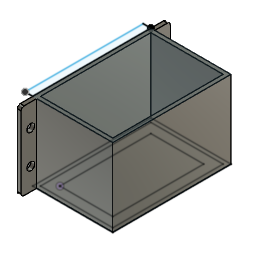
Housing_Power_Connector v1 (Autodesk Fusion 360 design; units mm, degrees)
Autodesk Fusion 360 part; units mm, degrees
sketch "Sketch1" plane through (0, 0, 0) normal (0, 0, 1) x (1, 0, 0)
  line L0 (0, 0) -> (27.2, 0)
  line L1 (27.2, 0) -> (27.2, 46.8)
  line L2 (27.2, 46.8) -> (0, 46.8)
  line L3 (0, 46.8) -> (0, 0)
  line L4 (-5, 51.8) -> (-5, -5)
  line L5 (-5, -5) -> (32.2, -5)
  line L6 (32.2, -5) -> (32.2, 51.8)
  line L7 (32.2, 51.8) -> (-5, 51.8)
  line L8 (-7, 53.8) -> (-7, -7)
  line L9 (-7, -7) -> (34.2, -7)
  line L10 (34.2, -7) -> (34.2, 53.8)
  line L11 (34.2, 53.8) -> (-7, 53.8)
  dimension "d1" = 27.2
  dimension "d2" = 46.8
  dimension "d3" = 5
  dimension "d4" = 7
  constraint horizontal L0
  constraint vertical L1
  constraint horizontal L2
  constraint vertical L3
  constraint coincident L0.start L3.end
  measures "d1" distance of L0.start L0.end
  measures "d2" distance of L0.start L2.end
extrude "Extrude1" add sketch "Sketch1" along normal blind 1.2 contours L4 L5 L6 L7
extrude "Extrude2" add sketch "Sketch1" along normal blind 40 contours L8 L9 L10 L11
sketch "Sketch2" plane through (0, 0, 40) normal (0, 0, 1) x (-1, 0, 0)
  line L0 (5, -51.8) -> (-32.2, -51.8)
  line L1 (-32.2, -51.8) -> (-32.2, 5)
  line L2 (-32.2, 5) -> (5, 5)
  line L3 (5, 5) -> (5, -51.8)
  line L4 (-34.2, -53.8) -> (7, -53.8)
  line L5 (7, -53.8) -> (7, 7)
  line L6 (7, 7) -> (-34.2, 7)
  line L7 (-34.2, 7) -> (-34.2, -53.8)
  line L8 (7, -53.8) -> (10.9437, -53.8)
  line L9 (10.9437, -53.8) -> (10.9437, 7)
  line L10 (10.9437, 7) -> (7, 7)
  line L11 (7, 7) -> (7, -53.8)
  constraint horizontal L8
  constraint vertical L9
  constraint horizontal L10
  constraint vertical L11
  constraint coincident L6 L9.end
  constraint coincident L4.end L5.start
sketch "Sketch3" plane through (0, -7, 0) normal (0, -1, 0) x (1, 0, 0)
  line L0 (-7, 0) -> (34.2, 0)
  line L1 (34.2, 0) -> (34.2, 40)
  line L2 (34.2, 40) -> (-7, 40)
  line L3 (-7, 40) -> (-7, 0)
  line L4 (-7, 0) -> (-5, 0)
  line L5 (-5, 0) -> (-5, 40)
  line L6 (-5, 40) -> (-7, 40)
  line L7 (-7, 40) -> (-7, 0)
  dimension "d9" = 2
  constraint horizontal L4
  constraint vertical L5
  constraint horizontal L6
  constraint vertical L7
  constraint coincident L2 L5.end
  constraint coincident L0.start L3.end
  measures "d9" distance of L0.start L4.end
extrude "Extrude3" add sketch "Sketch3" along normal blind 8 contours L0 L2 L3 L4 L5 L6 L7
sketch "Sketch4" plane through (0, 53.8, 0) normal (0, 1, 0) x (-1, 0, 0)
  line L0 (-34.2, 0) -> (7, 0)
  line L1 (7, 0) -> (7, 40)
  line L2 (7, 40) -> (-34.2, 40)
  line L3 (-34.2, 40) -> (-34.2, 0)
  line L4 (7, 0) -> (5, 0)
  line L5 (5, 0) -> (5, 40)
  line L6 (5, 40) -> (7, 40)
  line L7 (7, 40) -> (7, 0)
  dimension "d12" = 2
  constraint horizontal L4
  constraint vertical L5
  constraint horizontal L6
  constraint vertical L7
  constraint coincident L2 L5.end
  constraint coincident L0.end L1.start
  measures "d12" distance of L0.end L4.end
extrude "Extrude4" add sketch "Sketch4" along normal blind 8 contours L0 L1 L2 L4 L5 L6 L7
fillet "Fillet1" radius 1.5 4 edges at (-6, -15, 40) (-6, 61.8, 40) (-6, 61.8, 0) (-6, -15, 0)
sketch "Sketch5" plane through (-5, 0, 0) normal (1, 0, 0) x (0, 1, 0)
  arc A0 (60.3, 0) -> (61.8, 1.5) centre (60.3, 1.5) ccw
  line L0 (61.8, 1.5) -> (61.8, 38.5)
  arc A1 (61.8, 38.5) -> (60.3, 40) centre (60.3, 38.5) ccw
  line L1 (60.3, 40) -> (53.8, 40)
  line L2 (53.8, 40) -> (53.8, 0)
  line L3 (53.8, 0) -> (60.3, 0)
  line L4 (61.8, 11.3134) -> (-15, 11.3134) construction
  line L5 (61.8, 28.4248) -> (-15, 28.4248) construction
  line L6 (57.05, 0) -> (57.05, 40) construction
  line L7 (-10, 0) -> (-10, 40) construction
  circle A2 centre (57.05, 11.3134) radius 2
  circle A3 centre (57.05, 28.4248) radius 2
  circle A4 centre (-10, 11.3134) radius 2
  circle A5 centre (-10, 28.4248) radius 2
  dimension "d17" = 4
  dimension "d18" = 4
  dimension "d19" = 4
  dimension "d20" = 4
  constraint coincident L0 L4.start
  constraint perpendicular L0 L4
  constraint coincident L0 L5.start
  constraint perpendicular L0 L5
  constraint midpoint L3 L6.start
  constraint midpoint L1 L6.end
  constraint perpendicular L5 L7
  constraint coincident L6 A2.centre
  constraint coincident L4 A2.centre
  constraint coincident L6 A3.centre
  constraint coincident L5 A3.centre
  constraint coincident L7 A4.centre
  constraint coincident L4 A4.centre
  constraint coincident L7 A5.centre
  constraint coincident L5 A5.centre
  measures "d17" diameter of A2
  measures "d18" diameter of A3
  measures "d19" diameter of A4
  measures "d20" diameter of A5
extrude "Extrude5" cut sketch "Sketch5" against normal blind 4 contours A2 | A3 | A4 | A5
equation "d4 = 12 mm - 5 mm"
